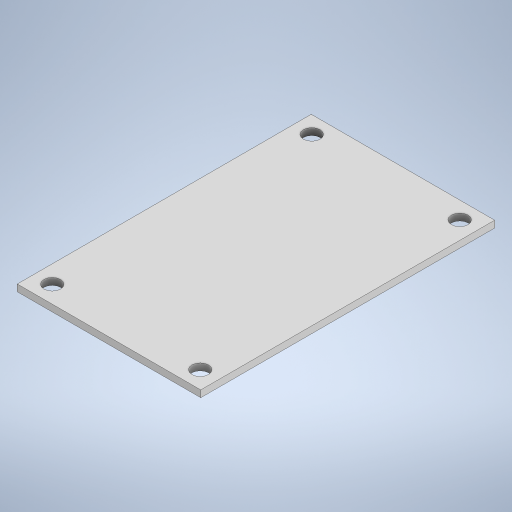
# Autodesk Inventor part: 降壓板
Saved by Autodesk Inventor 2024 (Build 280153000, 153)
## iProperties
Created: 2024-04-10
Part Number: 降壓板
Material: 一般
Document SubType Name: Modeling
Designer: rumse
Density: 1 g/cm^3
Appearance: 預設
Author: rumse
Autodesk Inventor part; units mm, degrees
ref_plane "YZ Plane" through (0, 0, 0) normal (1, 0, 0) x (0, 1, 0)
ref_plane "XZ Plane" through (0, 0, 0) normal (0, 1, 0) x (-1, 0, 0)
ref_plane "XY Plane" through (0, 0, 0) normal (0, 0, 1) x (1, 0, 0)
sketch "草圖1" plane through (0, 0, 0) normal (0, 1, 0) x (-1, 0, 0)
  line L0 (0, 0) -> (35.2, 0)
  line L1 (35.2, 0) -> (35.2, -56.4)
  line L2 (35.2, -56.4) -> (0, -56.4)
  line L3 (0, -56.4) -> (0, 0)
  line L4 (31.8, -3.3) -> (3.4, -3.3)
  line L5 (3.4, -3.3) -> (3.4, -53.1)
  line L6 (3.4, -53.1) -> (31.8, -53.1)
  line L7 (31.8, -53.1) -> (31.8, -3.3)
  circle A0 centre (31.8, -3.3) radius 1.6
  circle A1 centre (3.4, -3.3) radius 1.6
  circle A2 centre (31.8, -53.1) radius 1.6
  circle A3 centre (3.4, -53.1) radius 1.6
  dimension "d0" = 56.4
  dimension "d1" = 35.2
  dimension "d4" = 49.8
  dimension "d5" = 28.4
  dimension "d6" = 3.3
  dimension "d7" = 3.4
  dimension "d8" = 3.2
  dimension "d9" = 3.2
  dimension "d10" = 3.2
  dimension "d11" = 3.2
  constraints: 16 end point, 4 centre point, 4 coincident, 4 parallel, 2 horizontal, 2 perpendicular
  measures "d0" distance of L0.end L1.end
  measures "d1" distance of L1.end L2.end
  measures "d4" distance of L6.end L4.start
  measures "d5" distance of L5.end L6.end
  measures "d6" vertical distance of L0.start L4.end
  measures "d7" horizontal distance of L0.start L4.end
  measures "d8" diameter of A0
  measures "d9" diameter of A1
  measures "d10" diameter of A2
  measures "d11" diameter of A3
extrude "擠出1" add sketch "草圖1" along normal blind 1.3 contours L0 L1 L2 L3 | A1 L5 L4 | L4 L5 A1 | L4 A0 L7 A2 L6 A3 L5 A1 | A0 L7 L4 | L4 L7 A0 | A3 L6 L5 | L5 L6 A3 | A2 L6 L7 | L7 L6 A2
extrude "擠出2" cut sketch "草圖1" along normal blind 1.3 contours A1 L5 L4 | L4 L5 A1 | A0 L7 L4 | L4 L7 A0 | A3 L6 L5 | L5 L6 A3 | A2 L6 L7 | L7 L6 A2
